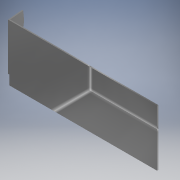
# Autodesk Inventor part: 15102898-16-P-0215
Saved by Autodesk Inventor 2017 (Build 210142000, 142)
## iProperties
Created: 2016-10-05
Part Number: 15102898-16-P-0215
Material: Aluminum 6061
Document SubType Name: Modeling
Designer: gus
Density: 2.7 g/cm^3
Appearance: Aluminum - Flat
Mass: 522.645 g
Surface Area: 1254.43 cm^2
Volume: 193.572 cm^3
Author: gus
Autodesk Inventor part; units mm, degrees
ref_plane "YZ Plane" through (0, 0, 0) normal (1, 0, 0) x (0, 1, 0)
ref_plane "XZ Plane" through (0, 0, 0) normal (0, 1, 0) x (-1, 0, 0)
ref_plane "XY Plane" through (0, 0, 0) normal (0, 0, 1) x (1, 0, 0)
sketch "Sketch1" plane through (0, 0, 0) normal (1, 0, 0) x (0, 1, 0)
  line L0 (0, 0) -> (-152.4, 0)
  line L1 (-152.4, 0) -> (-152.4, 3.175)
  line L2 (-152.4, 3.175) -> (0, 3.175)
  line L3 (0, 3.175) -> (0, 0)
  dimension "d0" = 152.4
  dimension "d1" = 3.175
  constraints: 8 end point, 2 parallel, 1 horizontal, 1 perpendicular
  measures "d0" distance of L1.end L2.end
  measures "d1" distance of L0.end L1.end
extrude "Extrusion1" add sketch "Sketch1" along normal blind 400.05
sketch "Sketch2" plane through (0, 0, 0) normal (-1, 0, 0) x (0, 0, 1)
  line L0 (0, 0) -> (3.175, 0) projected
  line L1 (3.175, 0) -> (-34.7333, 3.8172)
  line L2 (-34.7333, 3.8172) -> (-37.2781, -21.455)
  line L3 (-37.2781, -21.455) -> (-21.3975, -124.5257)
  line L4 (-21.3975, -124.5257) -> (3.175, -127)
  line L5 (3.175, -127) -> (3.175, 0)
  line L6 (0, -152.4) -> (0, 0) projected
  circle A0 centre (-8.255, -113.7628) radius 3.175
  line L7 (-21.3975, -124.5257) -> (3.175, -120.7397) construction
  line L8 (3.175, 0) -> (3.175, -152.4) projected
  circle A1 centre (-23.3696, -10.0913) radius 3.175
  dimension "d4" = 25.4
  dimension "d5" = 95.75
  dimension "d6" = 38.1
  dimension "d7" = 127
  dimension "d8" = 104.2869
  dimension "d9" = 6.35
  dimension "d11" = 11.43
  dimension "d12" = 8.636
  dimension "d15" = 12.7
  dimension "d16" = 6.35
  dimension "d17" = 12.7
  constraints: 12 end point, 2 centre point, 2 parallel, 2 perpendicular, 1 point on line
  measures "d4" distance of L1.end L2.end
  measures "d5" angle of L5 L1
  measures "d6" distance of L0.end L1.end
  measures "d7" distance of L4.end L0.end
  measures "d8" distance of L2.end L3.end
  measures "d9" diameter of A0
  measures "d11" distance from line of L5 A0.centre
  measures "d12" distance from line of L7 A0.centre
  measures "d15" distance from line of A1.centre L1
  measures "d16" diameter of A1
  measures "d17" distance from line of A1.centre L2
extrude "Extrusion3" add sketch "Sketch2" along normal blind 3.175
ref_plane "Work Plane1" through (200.025, 0, 0) normal (-1, 0, 0) x (0, 0, 1)
mirror "Mirror1" about plane through (200.025, 0, 0) normal (-1, 0, 0) of "Extrusion3"
body "Solid1"
